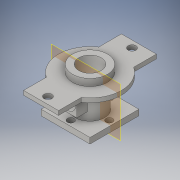
# Autodesk Inventor part: Vacuum Gripper holder
Saved by Autodesk Inventor 2016 (Build 200138000, 138)
## iProperties
Created: 2017-10-11
Part Number: Vacuum Gripper holder
Material: Generic
Document SubType Name: Modeling
Designer: ls769
Density: 1 g/cm^3
Appearance: Default
Author: ls769
Autodesk Inventor part; units mm, degrees
ref_plane "YZ Plane" through (0, 0, 0) normal (1, 0, 0) x (0, 1, 0)
ref_plane "XZ Plane" through (0, 0, 0) normal (0, 1, 0) x (-1, 0, 0)
sketch "Sketch1" plane through (0, 0, 0) normal (0, 0, 1) x (1, 0, 0)
  line L0 (12.525, 32) -> (8, 32)
  line L1 (8, 0) -> (8, 24)
  line L2 (22.5, 27) -> (22.5, 24)
  line L3 (22.5, 24) -> (12.525, 24)
  line L4 (10.5, 0) -> (10.5, 24)
  line L5 (10.5, 32) -> (8, 32)
  line L6 (8, 27) -> (8, 32)
  line L7 (12.525, 27) -> (22.5, 27)
  line L8 (8, 24) -> (8, 27)
  line L9 (12.525, 24) -> (10.5, 24)
  line L10 (12.525, 27) -> (12.525, 32)
  line L11 (8, 0) -> (10.5, 0)
  line L12 (0, -6.4) -> (0, 38.4) projected
  point P0 (0, 0)
  constraints: 24 end point, 3 parallel, 3 point on line, 2 horizontal, 2 perpendicular
revolve "Revolution1" add sketch "Sketch1" angle 360 about axis through (0, -10, 0) along (0, 1, 0)
sketch "Sketch2" plane through (0, 27, 0) normal (0, 1, 0) x (1, 0, 0)
  line L0 (12.5, 35) -> (-12.5, 35)
  line L1 (-12.5, 35) -> (-12.5, -35)
  line L2 (-12.5, -35) -> (12.5, -35)
  line L3 (12.5, -35) -> (12.5, 35)
  point P0 (0, 0)
  dimension "d8" = 25
  dimension "d9" = 70
  constraints: 8 end point, 2 parallel, 1 horizontal, 1 perpendicular
  measures "d8" distance of L2.end L1.end
  measures "d9" distance of L1.end L0.end
extrude "Extrusion1" add sketch "Sketch2" against normal blind 3
sketch "Sketch3" plane through (0, 27, 0) normal (0, 1, 0) x (1, 0, 0)
  circle A0 centre (0, 0) radius 8
  constraints: 1 centre point, 1 coincident
extrude "Extrusion2" cut sketch "Sketch3" against normal blind 3
sketch "Sketch4" plane through (-12.5, 27, 35) normal (0, 1, 0) x (1, 0, 0)
  line L0 (12.5, 35) -> (12.5, 65.078)
  line L1 (12.5, 35) -> (12.5, 4.922)
  circle A0 centre (12.5, 65.078) radius 2.8
  circle A1 centre (12.5, 4.922) radius 2.8
  dimension "d14" = 30.078
  dimension "d15" = 30.078
  dimension "d16" = 5.6
  dimension "d17" = 5.6
  constraints: 4 end point, 2 centre point, 2 coincident, 2 vertical
  measures "d14" distance of L0.start L0.end
  measures "d15" distance of L0.start L1.end
  measures "d16" diameter of A0
  measures "d17" diameter of A1
extrude "Extrusion3" cut sketch "Sketch4" against normal blind 3
sketch "Sketch5" plane through (0, 0, 0) normal (0, -1, 0) x (1, 0, 0)
  line L0 (17.5, 17.5) -> (-17.5, 17.5)
  line L1 (-17.5, 17.5) -> (-17.5, -17.5)
  line L2 (-17.5, -17.5) -> (17.5, -17.5)
  line L3 (17.5, -17.5) -> (17.5, 17.5)
  circle A0 centre (0, 13.8) radius 2.4
  circle A1 centre (13.8, 0) radius 2.4
  circle A2 centre (0, -13.8) radius 2.4
  circle A3 centre (-13.8, 0) radius 2.4
  point P0 (0, 0)
  dimension "d20" = 35
  dimension "d21" = 35
  dimension "d26" = 4.8
  dimension "d28" = 4.8
  constraints: 8 end point, 4 centre point, 2 parallel, 1 horizontal, 1 perpendicular
  measures "d20" distance of L2.end L1.end
  measures "d21" distance of L1.end L0.end
  measures "d26" diameter of A0
  measures "d28" diameter of A2
extrude "Extrusion4" add sketch "Sketch5" against normal blind 4.1
sketch "Sketch6" plane through (17.5, 0, -17.5) normal (0, 0, -1) x (-1, 0, 0)
  point P0 (17.5, 0)
ref_plane "Work Plane1" through (0, 0, 3) normal (0, 0, 1) x (1, 0, 0)
sketch "Sketch7" plane through (0, 0, 3) normal (0, 0, 1) x (1, 0, 0)
  line L0 (-10.5, 24) -> (10.5, 24) projected
  line L1 (6.5, 24) -> (-6.5, 24)
  line L2 (-6.5, 24) -> (-6.5, 10)
  line L3 (-6.5, 10) -> (6.5, 10)
  line L4 (6.5, 10) -> (6.5, 24)
  point P0 (0, 0)
  dimension "d33" = 13
  dimension "d34" = 14
  constraints: 8 end point, 2 parallel, 1 horizontal, 1 perpendicular, 1 point on line
  measures "d33" distance of L3.end L2.end
  measures "d34" distance of L2.end L1.end
extrude "Extrusion5" add sketch "Sketch7" along normal blind 13
sketch "Sketch8" plane through (0, 0, 16) normal (0, 0, 1) x (1, 0, 0)
  circle A0 centre (0, 17.1536) radius 5.75
  point P0 (0, 0)
  dimension "d37" = 11.5
  constraints: 1 centre point
  measures "d37" diameter of A0
extrude "Extrusion6" cut sketch "Sketch8" against normal blind 13
sketch "Sketch9" plane through (0, 4.1, 0) normal (0, 1, 0) x (1, 0, 0)
  circle A0 centre (0, 0) radius 8
  constraints: 1 centre point, 1 coincident
extrude "Extrusion7" add sketch "Sketch9" along normal blind 7.2
body "Solid1"
